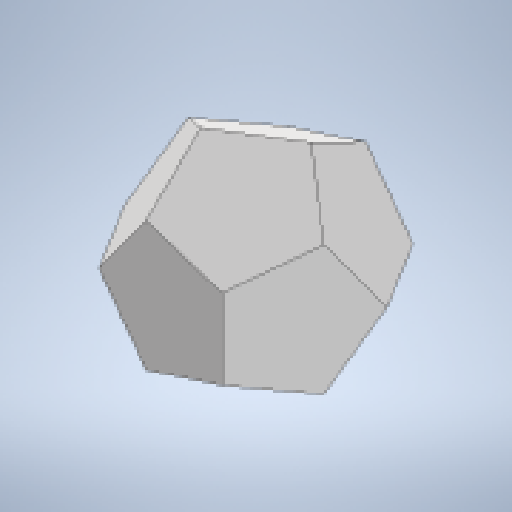
# Autodesk Inventor part: Dodecaedro
Saved by Autodesk Inventor 2024 (Build 280153000, 153)
## iProperties
Created: 2024-07-14
Part Number: Dodecaedro
Material: Genérico
Document SubType Name: Modeling
Designer: sergi
Density: 1 g/cm^3
Appearance: Valor por defecto
Author: sergi
Autodesk Inventor part; units mm, degrees
ref_plane "YZ Plane" through (0, 0, 0) normal (1, 0, 0) x (0, 1, 0)
ref_plane "XZ Plane" through (0, 0, 0) normal (0, 1, 0) x (-1, 0, 0)
ref_plane "XY Plane" through (0, 0, 0) normal (0, 0, 1) x (1, 0, 0)
sketch "Boceto2" plane through (0, 0, 0) normal (0, 0, 1) x (1, 0, 0)
  line L0 (-81.2065, -59) -> (-81.2065, 59)
  line L1 (-81.2065, 59) -> (31.0181, 95.464)
  line L2 (31.0181, 95.464) -> (100.3768, 0)
  line L3 (100.3768, 0) -> (31.0181, -95.464)
  line L4 (31.0181, -95.464) -> (-81.2065, -59)
  line L5 (0, 0) -> (-162.4131, 0)
  line L6 (-162.4131, 0) -> (-162.4131, 162.4131)
  line L7 (-162.4131, 162.4131) -> (0, 162.4131)
  line L8 (0, 162.4131) -> (0, 0)
  line L9 (-162.4131, 162.4131) -> (-81.2065, 0)
  dimension "d3" = 118
  dimension "d4" = 262.7899
  dimension "d5" = 26.565
  constraints: 20 end point, 2 midpoint, 2 parallel, 2 perpendicular, 1 coincident, 1 horizontal, 1 vertical, 11 other
  measures "d3" distance of L0.start L0.end
  measures "d4" distance from line of L2.end L6
  measures "d5" angle of L9 L0
extrude "Extrusión1" add sketch "Boceto2" along normal blind 262.7899 draft 26.57 contours L0 L5 L8 L1 L2 L3 L4 | L0 L1 L8 L5
sketch "Boceto3" plane through (0, 0, 262.7899) normal (0, 0, 1) x (1, 0, 0)
  line L0 (-31.0181, 95.464) -> (81.2065, 59)
  line L1 (81.2065, 59) -> (81.2065, -59)
  line L2 (81.2065, -59) -> (-31.0181, -95.464)
  line L3 (-31.0181, -95.464) -> (-100.3768, 0)
  line L4 (-100.3768, 0) -> (-31.0181, 95.464)
  point P0 (0, 0)
  point P1 (0, 0)
  dimension "d8" = 118
  constraints: 10 end point, 1 coincident, 1 vertical, 11 other
  measures "d8" distance of L1.end L2.end
extrude "Extrusión2" cut sketch "Boceto3" against normal blind 262.7899 draft 26.565 keep common part
ref_plane "Plano de trabajo1" through (-131.3998, -95.4675, 100.3648) normal (0.4910723, 0.3567849, 0.7947028) x (0.8506859, 0.0000184, -0.5256744)
feature "Dividir1" [suppressed]
ref_plane "Plano de trabajo2" through (31.0181, -95.464, 0) normal (-0.4910723, -0.3567849, -0.7947028) x (-0.8506859, -0.0000184, 0.5256744)
ref_plane "Plano de trabajo3" through (31.0181, -95.464, 0) normal (0.2628656, 0.809017, -0.5257311) x (-0.9510565, 0.309017, 0)
ref_plane "Plano de trabajo4" through (-81.2065, -59, 0) normal (-0.5877853, 0.809017, 0) x (-0.4253919, -0.3090653, 0.8506)
ref_plane "Plano de trabajo5" through (-81.2065, -59, 0) normal (0.8506508, 0, -0.5257311) x (0, 1, 0)
equation "\"d6\" = d4"
equation "\"d9\" = d4"
equation "\"d10\" = d5"
